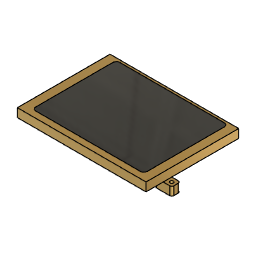
Rev4 v2 (Autodesk Fusion 360 archive; units mm, degrees)
design "RevEng TrackpadModule"
Autodesk Fusion 360 part; units mm, degrees
sketch "Sketch1" plane through (0, 0, 0) normal (0, 0, 1) x (1, 0, 0)
  line L0 (34.852, 42.8829) -> (-40.148, 42.8829)
  line L1 (-40.148, 42.8829) -> (-40.148, -11.1171)
  line L2 (-40.148, -11.1171) -> (34.852, -11.1171)
  line L3 (34.852, -11.1171) -> (34.852, 42.8829)
  line L4 (34.852, -11.1171) -> (34.852, -1.1171)
  line L5 (34.852, -1.1171) -> (38.652, -1.1171)
  line L6 (38.652, 3.8829) -> (34.852, 3.8829)
  line L7 (34.852, -1.1171) -> (38.652, -1.1171)
  line L8 (39.852, 0.0829) -> (39.852, 2.6829)
  line L9 (38.652, 3.8829) -> (34.852, 3.8829)
  line L10 (34.852, 3.8829) -> (34.852, -1.1171)
  circle A0 centre (37.352, 1.3829) radius 1
  arc A1 (38.652, -1.1171) -> (39.852, 0.0829) centre (38.652, 0.0829) ccw
  arc A2 (39.852, 2.6829) -> (38.652, 3.8829) centre (38.652, 2.6829) ccw
  line L11 (34.852, -1.1171) -> (31.052, -1.1171)
  line L12 (29.852, 0.0829) -> (29.852, 2.6829)
  line L13 (31.052, 3.8829) -> (34.852, 3.8829)
  line L14 (34.852, 3.8829) -> (34.852, -1.1171)
  arc A3 (29.852, 0.0829) -> (31.052, -1.1171) centre (31.052, 0.0829) ccw
  arc A4 (31.052, 3.8829) -> (29.852, 2.6829) centre (31.052, 2.6829) ccw
  line L15 (-2.648, 42.8829) -> (-2.648, -11.1171)
  line L16 (-2.648, 41.5829) -> (-33.148, 41.5829)
  line L17 (-2.648, 41.5829) -> (27.852, 41.5829)
  line L18 (29.852, 39.5829) -> (29.852, -5.4171)
  line L19 (27.852, -7.4171) -> (-31.9002, -7.4171)
  line L20 (-31.9002, -7.4171) -> (-33.148, -7.4171)
  line L21 (-35.148, -5.4171) -> (-35.148, 39.5829)
  arc A5 (27.852, -7.4171) -> (29.852, -5.4171) centre (27.852, -5.4171) ccw
  arc A6 (-35.148, -5.4171) -> (-33.148, -7.4171) centre (-33.148, -5.4171) ccw
  arc A7 (-33.148, 41.5829) -> (-35.148, 39.5829) centre (-33.148, 39.5829) ccw
  arc A8 (29.852, 39.5829) -> (27.852, 41.5829) centre (27.852, 39.5829) ccw
  point P0 (29.852, -1.1171)
  point P1 (-35.148, 41.5829)
  point P2 (29.852, 41.5829)
  point P3 (29.852, -7.4171)
  dimension "d1" = 75
  dimension "d2" = 54
  dimension "d5" = 10
  dimension "d8" = 5
  dimension "d9" = 2
  dimension "d10" = 1.2
  dimension "d11" = 5
  dimension "d12" = 1.2
  dimension "d13" = 5
  dimension "d14" = 5
  dimension "d15" = 1.2
  dimension "d18" = 32.5
  dimension "d19" = 49
  dimension "d20" = 1.3
  dimension "d21" = 2.5
  dimension "d22" = 2
  constraint horizontal L0
  constraint vertical L1
  constraint horizontal L2
  constraint vertical L3
  constraint perpendicular L2 L4
  constraint perpendicular L3 L5
  constraint coincident L3 L6.end
  constraint perpendicular L3 L6
  constraint horizontal L7
  constraint vertical L8
  constraint horizontal L9
  constraint vertical L10
  constraint tangent L8 A1
  constraint tangent L7 A1
  constraint tangent L9 A2
  constraint tangent L8 A2
  constraint horizontal L11
  constraint vertical L12
  constraint horizontal L13
  constraint vertical L14
  constraint coincident P0 L11
  constraint coincident P0 L12
  constraint tangent L11 A3
  constraint tangent L12 A3
  constraint tangent L12 A4
  constraint tangent L13 A4
  constraint equal A3 A4
  constraint midpoint L0 L15.start
  constraint midpoint L2 L15.end
  constraint coincident L15 L16.start
  constraint perpendicular L15 L16
  constraint perpendicular L15 L17
  constraint perpendicular L11 L18
  constraint perpendicular L15 L19
  constraint perpendicular L15 L20
  constraint perpendicular L16 L21
  constraint coincident P3 L18
  constraint coincident P3 L19
  constraint tangent L18 A5
  constraint tangent L19 A5
  constraint tangent L20 A6
  constraint tangent L21 A6
  constraint equal A5 A6
  constraint coincident P1 L16
  constraint coincident P1 L21
  constraint tangent L16 A7
  constraint tangent L21 A7
  constraint equal A5 A7
  constraint coincident P2 L17
  constraint coincident P2 L18
  constraint tangent L17 A8
  constraint tangent L18 A8
  constraint equal A5 A8
  measures "d1" distance of L0.start L0.end
  measures "d2" distance of L0.start L2.end
  measures "d5" distance of L2.end L4.end
  measures "d8" distance of L4.end L6.end
  measures "d9" diameter of A0
  measures "d10" radius of A1
  measures "d11" distance of L3 L8
  measures "d12" radius of A2
  measures "d13" distance of L4.end P0
  measures "d14" distance of L4.end L6.end
  measures "d15" radius of A3
  measures "d18" distance of L16.start P1
  measures "d19" distance of P2 P3
  measures "d20" distance of L0 L17
  measures "d21" distance of L8 A0.centre
  measures "d22" radius of A5
extrude "Extrude2" add sketch "Sketch1" against normal blind 5 contours L3 L5 L6 L7 L8 L9 L10 A1 A2 L14 | L3 L10 L11 L12 L13 L14 A3 A4 L18 makes body 1
extrude "Extrude1" add sketch "Sketch1" along normal blind 5 separate body contours L0 L3 L13 A4 L15 L17 L18 A8 | L0 L1 L2 L15 L16 L19 L20 L21 A6 A7 | L3 L10 L11 L12 L13 L14 A3 A4 L18 | L12 L15 L17 L18 L19 A5 A8 | L15 L16 L19 L20 L21 A6 A7 | L2 L3 L4 L11 A3 L15 L18 L19 A5 makes body 2
sketch "Sketch2" plane through (0, 0, 5) normal (0, 0, 1) x (-1, 0, 0)
  line L0 (-34.852, 11.1171) -> (-34.852, -42.8829)
  line L1 (-34.852, -42.8829) -> (40.148, -42.8829)
  line L2 (40.148, -42.8829) -> (40.148, 11.1171)
  line L3 (40.148, 11.1171) -> (-34.852, 11.1171)
sketch "Sketch3" plane through (0, 0, 5) normal (0, 0, 1) x (-1, 0, 0)
  line L0 (-29.852, -39.5829) -> (-29.852, 5.4171)
  line L1 (-27.852, 7.4171) -> (31.9002, 7.4171)
  arc A0 (-27.852, 7.4171) -> (-29.852, 5.4171) centre (-27.852, 5.4171) ccw
  arc A1 (35.148, 5.4171) -> (33.148, 7.4171) centre (33.148, 5.4171) ccw
  line L2 (31.9002, 7.4171) -> (33.148, 7.4171)
  line L3 (35.148, 5.4171) -> (35.148, -39.5829)
  arc A2 (33.148, -41.5829) -> (35.148, -39.5829) centre (33.148, -39.5829) ccw
  line L4 (2.648, -41.5829) -> (33.148, -41.5829)
  line L5 (2.648, -41.5829) -> (-27.852, -41.5829)
  arc A3 (-29.852, -39.5829) -> (-27.852, -41.5829) centre (-27.852, -39.5829) ccw
extrude "Extrude3" cut sketch "Sketch3" against normal blind 1 bodies 2
sketch "Sketch4" plane through (0, 0, 5) normal (0, 0, 1) x (-1, 0, 0)
sketch "Sketch5" plane through (0, 0, 4) normal (0, 0, 1) x (-1, 0, 0)
  arc A0 (-27.852, 7.4171) -> (-29.852, 5.4171) centre (-27.852, 5.4171) ccw
  line L0 (-29.852, 5.4171) -> (-29.852, -39.5829)
  arc A1 (-29.852, -39.5829) -> (-27.852, -41.5829) centre (-27.852, -39.5829) ccw
  line L1 (-27.852, -41.5829) -> (33.148, -41.5829)
  arc A2 (33.148, -41.5829) -> (35.148, -39.5829) centre (33.148, -39.5829) ccw
  line L2 (35.148, -39.5829) -> (35.148, 5.4171)
  arc A3 (35.148, 5.4171) -> (33.148, 7.4171) centre (33.148, 5.4171) ccw
  line L3 (33.148, 7.4171) -> (-27.852, 7.4171)
  line L4 (2.648, 7.4171) -> (2.648, -39.5791)
  line L5 (2.648, -37.5829) -> (-17.352, -37.5829)
  line L6 (2.648, -37.5829) -> (22.648, -37.5829)
  line L7 (22.648, -37.5829) -> (22.648, -7.5829)
  line L8 (22.648, -7.5829) -> (-17.352, -7.5829)
  line L9 (-17.352, -7.5829) -> (-17.352, -37.5829)
  dimension "d27" = 20
  dimension "d28" = 4
  dimension "d29" = 20
  dimension "d30" = 30
  constraint midpoint L3 L4.start
  constraint coincident L4 L5.start
  constraint perpendicular L4 L5
  constraint perpendicular L4 L6
  constraint perpendicular L6 L7
  constraint perpendicular L4 L8
  constraint perpendicular L5 L9
  measures "d27" distance of L5.start L5.end
  measures "d28" distance of L1 L5
  measures "d29" distance of L5.start L6.end
  measures "d30" distance of L6.end L7.end
extrude "Extrude4" cut sketch "Sketch5" against normal blind 60 contours L4 L6 L7 L8 | L4 L5 L8 L9 bodies 2
ref_plane "WorkPlane1" through (-2.648, 15.8829, 2.5) normal (-1, 0, 0) x (0, -1, 0)
mirror "Mirror1" about plane through (-2.648, 15.8829, 2.5) normal (-1, 0, 0) of bodies 1 makes body 3
copy_body "Body->Comp1" bodies 3 removing the originals makes body 4 in component "Component"
copy_body "Body->Comp2" bodies 1 removing the originals makes body 5 in component "Component'"
copy_body "Body->Comp3" bodies 2 removing the originals makes body 6 in component "MainBody"
sketch "Sketch6" plane through (0, 0, 5) normal (0, 0, 1) x (-1, 0, 0)
  line L0 (-29.852, -39.5829) -> (-29.852, 5.4171)
  arc A0 (-27.852, 7.4171) -> (-29.852, 5.4171) centre (-27.852, 5.4171) ccw
  line L1 (-27.852, 7.4171) -> (33.148, 7.4171)
  arc A1 (35.148, 5.4171) -> (33.148, 7.4171) centre (33.148, 5.4171) ccw
  line L2 (35.148, 5.4171) -> (35.148, -39.5829)
  arc A2 (33.148, -41.5829) -> (35.148, -39.5829) centre (33.148, -39.5829) ccw
  line L3 (33.148, -41.5829) -> (-27.852, -41.5829)
  arc A3 (-29.852, -39.5829) -> (-27.852, -41.5829) centre (-27.852, -39.5829) ccw
  line L4 (-34.852, 11.1171) -> (-34.852, -42.8829)
  line L5 (-34.852, -42.8829) -> (40.148, -42.8829)
  line L6 (40.148, -42.8829) -> (40.148, 11.1171)
  line L7 (40.148, 11.1171) -> (-34.852, 11.1171)
  line L8 (22.648, -7.5829) -> (22.648, -37.5829)
  line L9 (22.648, -37.5829) -> (-17.352, -37.5829)
  line L10 (-17.352, -37.5829) -> (-17.352, -7.5829)
  line L11 (-17.352, -7.5829) -> (22.648, -7.5829)
  arc A4 (-27.852, 7.4171) -> (-29.852, 5.4171) centre (-27.852, 5.4171) ccw
  line L12 (-29.852, 5.4171) -> (-29.852, -39.5829)
  arc A5 (-29.852, -39.5829) -> (-27.852, -41.5829) centre (-27.852, -39.5829) ccw
  line L13 (-27.852, -41.5829) -> (33.148, -41.5829)
  arc A6 (33.148, -41.5829) -> (35.148, -39.5829) centre (33.148, -39.5829) ccw
  line L14 (35.148, -39.5829) -> (35.148, 5.4171)
  arc A7 (35.148, 5.4171) -> (33.148, 7.4171) centre (33.148, 5.4171) ccw
  line L15 (33.148, 7.4171) -> (-27.852, 7.4171)
  line L16 (-34.852, -42.8829) -> (-34.852, 11.1171)
  line L17 (40.148, 11.1171) -> (-34.852, 11.1171)
  line L18 (40.148, 11.1171) -> (40.148, -42.8829)
  line L19 (-34.852, -42.8829) -> (40.148, -42.8829)
  line L20 (33.148, -41.5829) -> (-27.852, -41.5829)
  line L21 (-29.852, 5.4171) -> (-29.852, -39.5829)
  arc A8 (-29.852, -39.5829) -> (-27.852, -41.5829) centre (-27.852, -39.5829) ccw
  arc A9 (-27.852, 7.4171) -> (-29.852, 5.4171) centre (-27.852, 5.4171) ccw
  line L22 (-27.852, 7.4171) -> (33.148, 7.4171)
  arc A10 (35.148, 5.4171) -> (33.148, 7.4171) centre (33.148, 5.4171) ccw
  constraint coincident L4.end L5.start
  constraint coincident L4.start L7.end
  constraint coincident L6.end L7.start
  constraint coincident L5.end L6.start
  constraint coincident A2.start L3.start
  constraint coincident L3.end A3.end
  constraint coincident L0.end A0.end
  constraint coincident L0.start A3.start
  constraint tangent L13 A8
  constraint coincident A0.start L1.start
  constraint tangent L0 A9
  constraint coincident L1.end A1.end
  constraint coincident A1.start L2.start
  constraint tangent L15 A10
sketch "Sketch7" plane through (0, 0, 4) normal (0, 0, 1) x (-1, 0, 0)
  line L0 (22.648, -7.5829) -> (22.648, -37.5829)
  line L1 (22.648, -37.5829) -> (-17.352, -37.5829)
  line L2 (-17.352, -37.5829) -> (-17.352, -7.5829)
  line L3 (-17.352, -7.5829) -> (22.648, -7.5829)
  arc A0 (-27.852, 7.4171) -> (-29.852, 5.4171) centre (-27.852, 5.4171) ccw
  line L4 (-29.852, 5.4171) -> (-29.852, -39.5829)
  arc A1 (-29.852, -39.5829) -> (-27.852, -41.5829) centre (-27.852, -39.5829) ccw
  line L5 (-27.852, -41.5829) -> (33.148, -41.5829)
  arc A2 (33.148, -41.5829) -> (35.148, -39.5829) centre (33.148, -39.5829) ccw
  line L6 (35.148, -39.5829) -> (35.148, 5.4171)
  arc A3 (35.148, 5.4171) -> (33.148, 7.4171) centre (33.148, 5.4171) ccw
  line L7 (33.148, 7.4171) -> (-27.852, 7.4171)
extrude "Extrude1'" add sketch "Sketch7" along normal blind 1 separate body contours L0 L1 L2 L3 | A0 L4 A1 L5 A2 L6 A3 L7 makes body 7 in component "Component''"
component "Feet" placed x (1, 0, 0) y (0, 1, 0) z (0, 0, 1) at (0, 0, 0)
component "MainBody" placed x (1, 0, 0) y (0, 1, 0) z (0, 0, 1) at (0, 0, 0)
component "Component''" placed x (1, 0, 0) y (0, 1, 0) z (0, 0, 1) at (0, 0, 0)
component "Component'" placed x (1, 0, 0) y (0, 1, 0) z (0, 0, 1) at (0, 0, 0) in component "Feet"
component "Component" placed x (1, 0, 0) y (0, 1, 0) z (0, 0, 1) at (0, 0, 0) in component "Feet"
equation "d18 = ( 65 / 2 ) * 1 mm"
